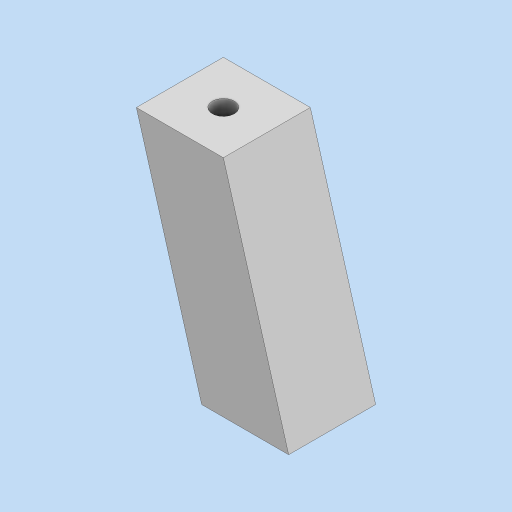
# Autodesk Inventor part: STRU_008_BilletBlock_Slanted
Saved by Autodesk Inventor 2024.3 (Build 283343000, 343)
## iProperties
Created: 2024-07-23
Part Number: STRU_008_BilletBlock_Slanted
Material: Generic
Document SubType Name: Modeling
Designer: bryan
Density: 1 g/cm^3
Appearance: Default
Author: bryan
Autodesk Inventor part; units mm, degrees
ref_plane "YZ Plane" through (0, 0, 0) normal (1, 0, 0) x (0, 1, 0)
ref_plane "XZ Plane" through (0, 0, 0) normal (0, 1, 0) x (-1, 0, 0)
ref_plane "XY Plane" through (0, 0, 0) normal (0, 0, 1) x (1, 0, 0)
sketch "Sketch1" plane through (0, 0, 0) normal (0, 1, 0) x (-1, 0, 0)
  line L0 (-9.525, -9.525) -> (9.525, -9.525)
  line L1 (9.525, -9.525) -> (9.525, 9.525)
  line L2 (9.525, 9.525) -> (-9.525, 9.525)
  line L3 (-9.525, 9.525) -> (-9.525, -9.525)
  line L4 (-9.525, -9.525) -> (9.525, 9.525) construction
  line L5 (9.525, -9.525) -> (-9.525, 9.525) construction
  point P0 (0, 0)
  dimension "d0" = 19.05
  dimension "d1" = 19.05
  constraints: 12 end point, 2 midpoint, 2 parallel, 1 horizontal, 1 perpendicular
  measures "d0" distance of L2.end L1.end
  measures "d1" distance of L1.end L0.end
sketch "Sketch2" plane through (0, 0, 0) normal (1, 0, 0) x (0, 1, 0)
  line L0 (0, 0) -> (112.776, 25.4)
  dimension "d2" = 112.776
  dimension "d3" = 25.4
  constraints: 2 end point
  measures "d2" horizontal distance of L0.start L0.end
  measures "d3" vertical distance of L0.start L0.end
sweep "Sweep1" add profiles "Sketch1" path "Sketch2"
sketch "Sketch3" plane through (-9.525, 112.776, 34.925) normal (0, 1, 0) x (1, 0, 0)
  line L0 (34.925, 76.2) -> (-15.875, 76.2)
  line L1 (-15.875, 76.2) -> (-15.875, -25.4)
  line L2 (-15.875, -25.4) -> (34.925, -25.4)
  line L3 (34.925, -25.4) -> (34.925, 76.2)
  line L4 (0, 25.4) -> (19.05, 25.4) projected
  line L5 (34.925, 76.2) -> (-15.875, -25.4) construction
  line L6 (-15.875, 76.2) -> (34.925, -25.4) construction
  point P0 (9.525, 34.925)
  point P1 (9.525, 25.4)
  dimension "d6" = 50.8
  dimension "d7" = 101.6
  constraints: 12 end point, 3 midpoint, 2 parallel, 1 horizontal, 1 perpendicular
  measures "d6" distance of L2.end L1.end
  measures "d7" distance of L1.end L0.end
extrude "Extrusion1" cut sketch "Sketch3" against normal blind 49.276
sketch "Sketch4" plane through (-9.525, 0, -9.525) normal (0, -1, 0) x (1, 0, 0)
  circle A0 centre (9.525, 9.525) radius 2.413
  dimension "d10" = 4.826
  constraints: 1 centre point, 1 coincident
  measures "d10" diameter of A0
extrude "Extrusion2" cut sketch "Sketch4" against normal blind 19.05
thread "Thread1"
sketch "Sketch5" plane through (-9.525, 63.5, 34.925) normal (0, 1, 0) x (1, 0, 0)
  circle A0 centre (9.525, 20.6232) radius 2.413
  line L0 (0, 11.0982) -> (0, 30.1482) projected
  line L1 (19.05, 11.0982) -> (0, 11.0982) projected
  point P0 (9.525, 34.925)
  point P1 (0, 20.6232)
  point P2 (9.525, 11.0982)
  dimension "d15" = 4.826
  constraints: 2 midpoint, 1 centre point, 1 horizontal alignment, 1 vertical alignment
  measures "d15" diameter of A0
extrude "Extrusion3" cut sketch "Sketch5" against normal blind 19.05
body "Solid1"
